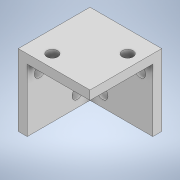
# Autodesk Inventor part: Ecken_Box
Saved by Autodesk Inventor 2021 (Build 250183000, 183)
## iProperties
Created: 2022-06-26
Part Number: Ecken_Box
Material: Generisch
Document SubType Name: Modeling
Designer: adria
Density: 1 g/cm^3
Appearance: Vorgabe
Mass: 20.2483 g
Surface Area: 98.2422 cm^2
Volume: 20.2483 cm^3
Author: adria
Autodesk Inventor part; units mm, degrees
ref_plane "YZ Plane" through (0, 0, 0) normal (1, 0, 0) x (0, 1, 0)
ref_plane "XZ Plane" through (0, 0, 0) normal (0, 1, 0) x (-1, 0, 0)
ref_plane "XY Plane" through (0, 0, 0) normal (0, 0, 1) x (1, 0, 0)
sketch "Skizze1" plane through (0, 0, 0) normal (0, 0, 1) x (1, 0, 0)
  line L0 (-20, -20) -> (20, -20)
  line L1 (20, -20) -> (20, 20)
  line L2 (20, 20) -> (-20, 20)
  line L3 (-20, 20) -> (-20, -20)
  line L4 (-20, -20) -> (20, 20) construction
  line L5 (20, -20) -> (-20, 20) construction
  point P0 (0, 0)
  dimension "d0" = 40
  dimension "d1" = 40
  constraints: 12 end point, 2 midpoint, 2 parallel, 1 horizontal, 1 perpendicular
  measures "d0" distance of L2.end L1.end
  measures "d1" distance of L1.end L0.end
extrude "Extrusion1" add sketch "Skizze1" along normal blind 5
sketch "Skizze2" plane through (-20, -20, 0) normal (-1, 0, 0) x (0, 0, 1)
  line L0 (5, 40) -> (5, 0) projected
  line L1 (0, 0) -> (40, 0)
  line L2 (40, 0) -> (40, 40)
  line L3 (40, 40) -> (0, 40)
  line L4 (0, 40) -> (0, 0)
  point P0 (0, 20)
  dimension "d4" = 40
  dimension "d5" = 40
  constraints: 8 end point, 2 parallel, 1 horizontal, 1 perpendicular
  measures "d4" distance of L3.end L2.end
  measures "d5" distance between parallel lines of L1 L3
extrude "Extrusion2" add sketch "Skizze2" against normal blind 5 contours L3 L2 L1 L0
sketch "Skizze3" plane through (-20, 20, 0) normal (0, 1, 0) x (1, 0, 0)
  line L0 (40, 0) -> (0, 0) projected
  line L1 (0, 0) -> (0, -40) projected
  line L2 (5, -5) -> (5, -40) projected
  line L3 (40, -5) -> (5, -5) projected
  line L4 (0, 0) -> (40, 0)
  line L5 (40, 0) -> (40, -40)
  line L6 (40, -40) -> (0, -40)
  line L7 (0, -40) -> (0, 0)
  point P0 (20, 0)
  point P1 (5, -40)
  point P2 (0, -5)
  dimension "d8" = 40
  dimension "d9" = 40
  constraints: 8 end point, 2 parallel, 1 horizontal, 1 perpendicular
  measures "d8" distance between parallel lines of L0 L6
  measures "d9" distance between parallel lines of L1 L5
extrude "Extrusion3" add sketch "Skizze3" against normal blind 5 contours L5 L6 L2 L3
sketch "Skizze4" plane through (-15, -20, 0) normal (1, 0, 0) x (0, 0, -1)
  line L0 (-5, 35) -> (-40, 35) projected
  line L1 (-40, 40) -> (-40, 0) projected
  line L2 (-40, 0) -> (-5, 0) projected
  line L3 (-5, 40) -> (-5, 0) projected
  point P0 (0, 20)
  point P1 (-33, 28)
  point P2 (-12, 7)
  dimension "d12" = 7
  dimension "d13" = 7
  dimension "d14" = 7
  dimension "d15" = 7
  measures "d12" distance from line of L1 point (-33, 28)
  measures "d13" distance from line of L0 point (-33, 28)
  measures "d14" distance from line of L3 point (-12, 7)
  measures "d15" distance from line of L2 point (-12, 7)
hole "Bohrung1" at (-15, 8, 33) at (-15, -13, 12) direction (-1, 0, 0) diameter 6.1 end through all
sketch "Skizze5" plane through (-20, 15, 0) normal (0, -1, 0) x (1, 0, 0)
  line L0 (40, 5) -> (40, 40) projected
  line L1 (40, 40) -> (5, 40) projected
  line L2 (5, 5) -> (5, 40) projected
  line L3 (40, 5) -> (5, 5) projected
  point P0 (20, 0)
  point P1 (12, 33)
  point P2 (33, 12)
  dimension "d23" = 7
  dimension "d24" = 7
  dimension "d25" = 7
  dimension "d26" = 7
  measures "d23" distance from line of L1 point (12, 33)
  measures "d24" distance from line of L2 point (12, 33)
  measures "d25" distance from line of L0 point (33, 12)
  measures "d26" distance from line of L3 point (33, 12)
hole "Bohrung2" at (-8, 15, 33) at (13, 15, 12) direction (0, 1, 0) diameter 6.1 end through all
sketch "Skizze6" plane through (0, 0, 5) normal (0, 0, 1) x (1, 0, 0)
  line L0 (20, 15) -> (-15, 15) projected
  line L1 (-15, 15) -> (-15, -20) projected
  line L2 (-15, -20) -> (20, -20) projected
  line L3 (20, -20) -> (20, 15) projected
  point P0 (0, 0)
  point P1 (-8, -13)
  point P2 (13, 8)
  dimension "d34" = 7
  dimension "d35" = 7
  dimension "d36" = 7
  dimension "d37" = 7
  measures "d34" distance from line of L2 point (-8, -13)
  measures "d35" distance from line of L1 point (-8, -13)
  measures "d36" distance from line of L3 point (13, 8)
  measures "d37" distance from line of L0 point (13, 8)
hole "Bohrung3" at (-8, -13, 5) at (13, 8, 5) direction (0, 0, -1) diameter 6.1 end through all
equation "\"d5\" = d4"
equation "\"d8\" = d9"
equation "\"d13\" = d12"
equation "\"d14\" = d12"
equation "\"d15\" = d12"
equation "\"d24\" = d23"
equation "\"d25\" = d23"
equation "\"d26\" = d23"
equation "\"d35\" = d34"
equation "\"d36\" = d34"
equation "\"d37\" = d34"
